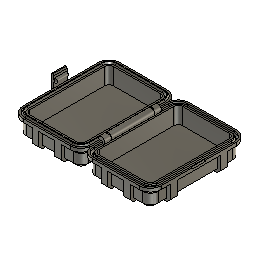
Parametric_Rugged_Box (Autodesk Fusion 360 design; units mm, degrees)
Autodesk Fusion 360 part; units mm, degrees
note: some values were not read from the file. Chosen so that the rebuilt part matches the saved one: where a step starts; which pieces of a blend or face edit are solid. Set by a fixed rule: which sketch regions a step uses.
sketch "Base Sketch" plane through (0, 0, 0) normal (0, 0, 1) x (1, 0, 0)
  line L0 (4, 0) -> (46, 0)
  line L1 (50, 4) -> (50, 71)
  line L2 (46, 75) -> (4, 75)
  line L3 (0, 71) -> (0, 4)
  arc A0 (46, 0) -> (50, 4) centre (46, 4) ccw
  arc A1 (50, 71) -> (46, 75) centre (46, 71) ccw
  arc A2 (4, 75) -> (0, 71) centre (4, 71) ccw
  arc A3 (0, 4) -> (4, 0) centre (4, 4) ccw
  point P0 (50, 0)
  point P1 (0, 75)
  dimension "d6" = 50
  dimension "d7" = 75
  dimension "d8" = 4
  constraint horizontal L0
  constraint vertical L1
  constraint horizontal L2
  constraint vertical L3
  constraint coincident P0 L0
  constraint coincident P0 L1
  constraint tangent L0 A0
  constraint tangent L1 A0
  constraint tangent L1 A1
  constraint tangent L2 A1
  constraint equal A0 A1
  constraint coincident P1 L2
  constraint coincident P1 L3
  constraint tangent L2 A2
  constraint tangent L3 A2
  constraint equal A0 A2
  constraint coincident origin L0
  constraint coincident origin L3
  constraint tangent L0 A3
  constraint tangent L3 A3
  constraint equal A0 A3
  measures "d6" distance of origin P0
  measures "d7" distance of origin P1
  measures "d8" radius of A0
ref_plane "WorkPlane1" through (0, 37.5, 0) normal (0, 1, 0) x (0, 0, 1)
sketch "Top Sketch" plane through (0, 37.5, 0) normal (0, 1, 0) x (1, 0, 0)
  line L0 (0, 0) -> (-3, 0)
  line L1 (-3, 0) -> (-3, -15)
  line L2 (-3, -15) -> (0, -15)
  line L3 (0, -15) -> (0, 0)
  line L4 (-3, -15) -> (-6, -15)
  line L5 (-6, -15) -> (-6, -12)
  line L6 (-6, -12) -> (-3, -12)
  line L7 (-3, -12) -> (-3, -15)
  line L8 (0, 0) -> (25, 0)
  line L9 (25, 0) -> (25, 3)
  line L10 (25, 3) -> (0, 3)
  line L11 (0, 3) -> (0, 0)
  line L12 (0, 3) -> (-3, 0)
  line L13 (-6, -12) -> (-3, -9)
  line L14 (-4.5, -15) -> (-3.3536, -16.1464)
  line L15 (-4.5, -15) -> (-2.3787, -15) construction
  line L16 (-2.6464, -16.1464) -> (-1.5, -15)
  arc A0 (-3.3536, -16.1464) -> (-2.6464, -16.1464) centre (-3, -15.7929) ccw
  dimension "d12" = 3
  dimension "d13" = 15
  dimension "d14" = 3
  dimension "d15" = 3
  dimension "d16" = 25
  dimension "d17" = 3
  dimension "d97" = 45
  dimension "d146" = 0.5
  dimension "d284" = 45
  constraint horizontal L0
  constraint vertical L1
  constraint horizontal L2
  constraint vertical L3
  constraint coincident L0.start L3.end
  constraint horizontal L4
  constraint vertical L5
  constraint horizontal L6
  constraint vertical L7
  constraint horizontal L8
  constraint vertical L9
  constraint horizontal L10
  constraint vertical L11
  constraint coincident L1 L13.end
  constraint parallel L12 L13
  constraint horizontal L15
  constraint midpoint L4 L14.start
  constraint midpoint L2 L16.end
  constraint tangent L14 A0
  constraint tangent L16 A0
  measures "d12" distance of L0.start L0.end
  measures "d13" distance of L0.start L2.end
  measures "d14" distance of L1.end L4.end
  measures "d15" distance of L1.end L6.end
  measures "d16" distance of L0.start L8.end
  measures "d17" distance of L0.start L10.end
  measures "d97" angle of L14 L15
  measures "d146" radius of A0
  measures "d284" angle of L2 L16
sweep "Sweep1" add profiles "Top Sketch" path "Base Sketch" along L0 A0 L1 A1 L2 A2 L3 A3 section 1 contours L0 L1 L2 L3 L7 | L8 L9 L10 L11 | L0 L11 L12 | L1 L6 L13 | L1 L4 L5 L6 L7 makes body 1
sketch "Bottom Sketch" plane through (0, 37.5, 0) normal (0, 1, 0) x (1, 0, 0)
  line L0 (0, 0) -> (-3, 0)
  line L1 (-3, 0) -> (-3, -15)
  line L2 (-3, -15) -> (0, -15)
  line L3 (0, -15) -> (0, 0)
  line L4 (0, 0) -> (25, 0)
  line L5 (25, 0) -> (25, 3)
  line L6 (25, 3) -> (0, 3)
  line L7 (0, 3) -> (0, 0)
  line L8 (-3, -15) -> (-6, -15)
  line L9 (-6, -15) -> (-6, -12)
  line L10 (-6, -12) -> (-3, -12)
  line L11 (-3, -12) -> (-3, -15)
  line L12 (0, 3) -> (-3, 0)
  line L13 (-6, -12) -> (-3, -9)
  line L14 (-4.5, -15) -> (-1.5, -15)
  line L15 (-1.5, -15) -> (-1.5, -12)
  line L16 (-1.5, -12) -> (-4.5, -12)
  line L17 (-4.5, -12) -> (-4.5, -15)
  line L18 (-3.3536, -12.3536) -> (-4.5, -13.5)
  line L19 (-2.6464, -12.3536) -> (-1.5, -13.5)
  arc A0 (-2.6464, -12.3536) -> (-3.3536, -12.3536) centre (-3, -12.7071) ccw
  dimension "d24" = 3
  dimension "d25" = 15
  dimension "d26" = 25
  dimension "d27" = 3
  dimension "d28" = 3
  dimension "d29" = 3
  dimension "d90" = 3
  dimension "d145" = 0.5
  constraint horizontal L0
  constraint vertical L1
  constraint horizontal L2
  constraint vertical L3
  constraint coincident L0.start L3.end
  constraint horizontal L4
  constraint vertical L5
  constraint horizontal L6
  constraint vertical L7
  constraint horizontal L8
  constraint vertical L9
  constraint horizontal L10
  constraint vertical L11
  constraint coincident L1 L13.end
  constraint parallel L12 L13
  constraint horizontal L14
  constraint vertical L15
  constraint horizontal L16
  constraint vertical L17
  constraint midpoint L8 L14.start
  constraint midpoint L17 L18.end
  constraint midpoint L15 L19.end
  constraint perpendicular L18 L19
  constraint coincident L10.end L18
  constraint coincident L10.end L19
  constraint tangent L18 A0
  constraint tangent L19 A0
  measures "d24" distance of L0.start L0.end
  measures "d25" distance of L0.start L2.end
  measures "d26" distance of L0.start L4.end
  measures "d27" distance of L0.start L6.end
  measures "d28" distance of L1.end L8.end
  measures "d29" distance of L1.end L10.end
  measures "d90" distance of L14.start L16.end
  measures "d145" radius of A0
sweep "Sweep2" add profiles "Bottom Sketch" path "Base Sketch" along L0 A0 L1 A1 L2 A2 L3 A3 section 1 separate body makes body 2
ref_plane "WorkPlane2" through (0, 18, 0) normal (0, 1, 0) x (0, 0, 1)
sketch "Rib Bottom" plane through (0, 18, 0) normal (0, 1, 0) x (1, 0, 0)
  line L0 (0, 0) -> (-6, 0)
  line L1 (-6, 0) -> (-6, -15)
  line L2 (-6, -15) -> (0, -15)
  line L3 (0, -15) -> (0, 0)
  line L4 (0, 0) -> (25, 0)
  line L5 (25, 0) -> (25, 3)
  line L6 (25, 3) -> (0, 3)
  line L7 (0, 3) -> (0, 0)
  line L8 (0, 0) -> (-3, 0)
  line L9 (-3, 0) -> (-3, 3)
  line L10 (-3, 3) -> (0, 3)
  line L11 (0, 3) -> (0, 0)
  line L12 (-3, 3) -> (-6, 0)
  dimension "d37" = 6
  dimension "d38" = 15
  dimension "d39" = 25
  dimension "d40" = 3
  dimension "d41" = 3
  dimension "d42" = 3
  constraint horizontal L0
  constraint vertical L1
  constraint horizontal L2
  constraint vertical L3
  constraint coincident L0.start L3.end
  constraint horizontal L4
  constraint vertical L5
  constraint horizontal L6
  constraint vertical L7
  constraint horizontal L8
  constraint vertical L9
  constraint horizontal L10
  constraint vertical L11
  measures "d37" distance of L0.start L0.end
  measures "d38" distance of L0.start L2.end
  measures "d39" distance of L0.start L4.end
  measures "d40" distance of L0.start L6.end
  measures "d41" distance of L0.start L8.end
  measures "d42" distance of L0.start L6.end
extrude "Extrude1" add sketch "Rib Bottom" against normal blind 6 bodies 2
ref_plane "WorkPlane3" through (0, 57, 0) normal (0, 1, 0) x (0, 0, 1)
extrude "Extrude2" add sketch "Rib Bottom" along normal blind 6 from surface at 39 bodies 2
ref_plane "WorkPlane4" through (25, 0, 0) normal (1, 0, 0) x (0, 1, 0)
mirror "Mirror1" about plane through (25, 0, 0) normal (1, 0, 0) of "Extrude1", "Extrude2"
sketch "Rib Top" plane through (0, 37.5, 0) normal (0, 1, 0) x (1, 0, 0)
  line L0 (0, 0) -> (-6, 0)
  line L1 (-6, 0) -> (-6, -15)
  line L2 (-6, -15) -> (0, -15)
  line L3 (0, -15) -> (0, 0)
  line L4 (0, 0) -> (25, 0)
  line L5 (25, 0) -> (25, 3)
  line L6 (25, 3) -> (0, 3)
  line L7 (0, 3) -> (0, 0)
  line L8 (0, 0) -> (-3, 0)
  line L9 (-3, 0) -> (-3, 3)
  line L10 (-3, 3) -> (0, 3)
  line L11 (0, 3) -> (0, 0)
  line L12 (-3, 3) -> (-6, 0)
  dimension "d52" = 6
  dimension "d53" = 15
  dimension "d54" = 25
  dimension "d55" = 3
  dimension "d56" = 3
  dimension "d57" = 3
  constraint horizontal L0
  constraint vertical L1
  constraint horizontal L2
  constraint vertical L3
  constraint coincident L0.start L3.end
  constraint horizontal L4
  constraint vertical L5
  constraint horizontal L6
  constraint vertical L7
  constraint horizontal L8
  constraint vertical L9
  constraint horizontal L10
  constraint vertical L11
  measures "d52" distance of L0.start L0.end
  measures "d53" distance of L0.start L2.end
  measures "d54" distance of L0.start L4.end
  measures "d55" distance of L0.start L6.end
  measures "d56" distance of L0.start L8.end
  measures "d57" distance of L0.start L6.end
extrude "Extrude3" add sketch "Rib Top" against normal blind 6 from surface at -19.5 bodies 1
extrude "Extrude4" add sketch "Rib Top" along normal blind 6 from surface at 19.5 bodies 1
mirror "Mirror2" about plane through (25, 0, 0) normal (1, 0, 0) of "Extrude3", "Extrude4"
ref_plane "WorkPlane5" through (18, 0, 0) normal (1, 0, 0) x (0, 1, 0)
ref_plane "WorkPlane6" through (32, 0, 0) normal (1, 0, 0) x (0, 1, 0)
sketch "Rib Wid" plane through (18, 0, 0) normal (1, 0, 0) x (0, 1, 0)
  line L0 (0, 0) -> (-6, 0)
  line L1 (-6, 0) -> (-6, 15)
  line L2 (-6, 15) -> (0, 15)
  line L3 (0, 15) -> (0, 0)
  line L4 (0, 0) -> (37.5, 0)
  line L5 (37.5, 0) -> (37.5, -3)
  line L6 (37.5, -3) -> (0, -3)
  line L7 (0, -3) -> (0, 0)
  line L8 (0, 0) -> (-3, 0)
  line L9 (-3, 0) -> (-3, -3)
  line L10 (-3, -3) -> (0, -3)
  line L11 (0, -3) -> (0, 0)
  line L12 (-3, -3) -> (-6, 0)
  line L13 (0, -3) -> (-6, -3)
  line L14 (-6, -3) -> (-6, 12)
  line L15 (-6, 12) -> (0, 12)
  line L16 (0, 12) -> (0, -3)
  dimension "d68" = 6
  dimension "d69" = 15
  dimension "d70" = 37.5
  dimension "d71" = 3
  dimension "d72" = 3
  dimension "d73" = 3
  dimension "d74" = 6
  dimension "d75" = 15
  constraint horizontal L0
  constraint vertical L1
  constraint horizontal L2
  constraint vertical L3
  constraint coincident L0.start L3.end
  constraint horizontal L4
  constraint vertical L5
  constraint horizontal L6
  constraint vertical L7
  constraint horizontal L8
  constraint vertical L9
  constraint horizontal L10
  constraint vertical L11
  constraint horizontal L13
  constraint vertical L14
  constraint horizontal L15
  constraint vertical L16
  measures "d68" distance of L0.start L0.end
  measures "d69" distance of L0.start L2.end
  measures "d70" distance of L0.start L4.end
  measures "d71" distance of L0.start L6.end
  measures "d72" distance of L0.start L8.end
  measures "d73" distance of L0.start L6.end
  measures "d74" distance of L6.end L13.end
  measures "d75" distance of L6.end L15.end
extrude "Extrude5" add sketch "Rib Wid" against normal blind 6 contours L0 L7 L8 L9 L10 L11 L13 L16 | L0 L1 L3 L8 L14 L15 L16 | L4 L5 L6 L7 L11 L16 | L0 L9 L12 | L1 L2 L3 L15 bodies 2
extrude "Extrude6" add sketch "Rib Wid" along normal blind 6 from surface at 14 contours L0 L7 L8 L9 L10 L11 L13 L16 | L0 L1 L3 L8 L14 L15 L16 | L4 L5 L6 L7 L11 L16 | L0 L9 L12 | L1 L2 L3 L15 bodies 2
ref_plane "WorkPlane7" through (25, 37.5, 4.5) normal (0, -1, 0) x (0, 0, -1)
mirror "Mirror3" about plane through (25, 37.5, 4.5) normal (0, -1, 0) of "Extrude5", "Extrude6"
extrude "Extrude7" add sketch "Rib Wid" against normal blind 6 contours L0 L7 L8 L9 L10 L11 L13 L16 | L0 L1 L3 L8 L14 L15 L16 | L4 L5 L6 L7 L11 L16 | L0 L9 L12 bodies 1
extrude "Extrude8" add sketch "Rib Wid" along normal blind 6 from surface at 14 contours L0 L7 L8 L9 L10 L11 L13 L16 | L0 L1 L3 L8 L14 L15 L16 | L4 L5 L6 L7 L11 L16 | L0 L9 L12 bodies 1
mirror "Mirror4" about plane through (25, 37.5, 4.5) normal (0, -1, 0) of "Extrude7", "Extrude8"
sweep "Sweep3" cut profiles "Bottom Sketch" path "Base Sketch" along L0 A0 L1 A1 L2 A2 L3 A3 section 1 contours L1 L2 L11 L14 L15 L19 A0 | L1 L8 L11 L14 L17 L18 A0 bodies 2
sweep "Sweep4" add profiles "Top Sketch" path "Base Sketch" along L0 A0 L1 A1 L2 A2 L3 A3 section 1 contours L2 L4 L14 L16 A0 bodies 1
sketch "Hinge" plane through (0, 0, 0) normal (0, 1, 0) x (1, 0, 0)
  line L0 (0, 0) -> (-6, 0) construction
  line L1 (-6, 0) -> (-6, -15) construction
  line L2 (-6, -15) -> (0, -15) construction
  line L3 (0, -15) -> (0, 0) construction
  circle A0 centre (-6, -15) radius 3
  circle A1 centre (-6, -15) radius 1.5
  circle A2 centre (-6, -15) radius 3.1
  line L4 (-6, -15) -> (-4.5, -15)
  line L5 (-4.5, -15) -> (-4.5, -18)
  line L6 (-4.5, -18) -> (-6, -18)
  line L7 (-6, -18) -> (-6, -15)
  line L8 (-6, -15) -> (-7.5, -15)
  line L9 (-7.5, -15) -> (-7.5, -18)
  line L10 (-7.5, -18) -> (-6, -18)
  line L11 (-6, -18) -> (-6, -15)
  line L12 (0, 0) -> (-6, 0) construction
  line L13 (-6, 0) -> (-6, -15) construction
  line L14 (-6, -15) -> (0, -15) construction
  line L15 (0, -15) -> (0, 0) construction
  circle A3 centre (-6, -15) radius 3
  circle A4 centre (-6, -15) radius 3.2
  dimension "d329" = 6
  dimension "d330" = 15
  dimension "d331" = 6
  dimension "d332" = 3
  dimension "d339" = 6.2
  dimension "d345" = 1.5
  dimension "d346" = 3
  dimension "d347" = 1.5
  dimension "d348" = 3
  dimension "d355" = 6
  dimension "d356" = 15
  dimension "d357" = 6
  dimension "d358" = 0.2
  constraint horizontal L0
  constraint vertical L1
  constraint horizontal L2
  constraint vertical L3
  constraint coincident L0.start L3.end
  constraint coincident L1.end L2.start
  constraint concentric A0 A1
  constraint concentric A0 A2
  constraint horizontal L4
  constraint vertical L5
  constraint horizontal L6
  constraint vertical L7
  constraint horizontal L8
  constraint vertical L9
  constraint horizontal L10
  constraint vertical L11
  constraint horizontal L12
  constraint vertical L13
  constraint horizontal L14
  constraint vertical L15
  measures "d329" distance of L0.start L0.end
  measures "d330" distance of L0.start L2.end
  measures "d331" diameter of A0
  measures "d332" diameter of A1
  measures "d339" diameter of A2
  measures "d345" distance of L1.end L4.end
  measures "d346" distance of L1.end L6.end
  measures "d347" distance of L1.end L8.end
  measures "d348" distance of L1.end L6.end
  measures "d355" distance of L0.start L0.end
  measures "d356" distance of L0.start L2.end
  measures "d357" diameter of A3
extrude "Extrude58" add sketch "Hinge" along normal up to surface (6 mm away) from surface at 12 contours A0 A1 L5 L9 A3 | A0 A1 L7 L9 L11 A3 | A0 A1 L5 L7 L11 A3 | A1 L7 L8 L11 | A1 L4 L8 | A1 L4 L7 L11 bodies 1
extrude "Extrude59" add sketch "Hinge" along normal up to surface (6 mm away) from surface at 57 contours A0 A1 L5 L9 A3 | A0 A1 L7 L9 L11 A3 | A0 A1 L5 L7 L11 A3 | A1 L7 L8 L11 | A1 L4 L8 | A1 L4 L7 L11 bodies 1
extrude "Extrude60" cut sketch "Hinge" along normal up to surface (39 mm away) from surface at 18 contours A0 A1 L5 L9 A3 | A0 A2 L5 L9 A3 | A0 A1 L7 L9 L11 A3 | A0 A2 L9 L10 A3 | A0 A2 L5 L6 A3 | A0 A1 L5 L7 L11 A3 | A2 L6 L10 | A1 L7 L8 L11 | A1 L4 L8 | A1 L4 L7 L11 bodies 1
extrude "Extrude61" cut sketch "Hinge" against normal blind 0.8 from surface at 18 contours A0 A1 L7 L9 L11 A3 | A0 A1 L5 L7 L11 A3 | A1 L7 L8 L11 | A1 L4 L7 L11 bodies 1
extrude "Extrude62" cut sketch "Hinge" along normal blind 0.8 from surface at 57 contours A0 A1 L7 L9 L11 A3 | A0 A1 L5 L7 L11 A3 | A1 L7 L8 L11 | A1 L4 L7 L11 bodies 1
extrude "Extrude63" cut sketch "Hinge" along normal up to surface (6.4 mm away) from surface at 11.8 contours A0 A1 L5 L9 A3 | A0 A2 L5 L9 A3 | A0 A1 L7 L9 L11 A3 | A0 A2 L9 L10 A3 | A0 A2 L5 L6 A3 | A0 A1 L5 L7 L11 A3 | A2 L6 L10 | A1 L7 L8 L11 | A1 L4 L8 | A2 L5 L9 A4 | A2 L9 L10 A4 | A1 L4 L7 L11 | A2 L5 L6 A4 | A2 L6 L10 A4 bodies 2
extrude "Extrude64" cut sketch "Hinge" along normal up to surface (6.4 mm away) from surface at 56.8 contours A0 A1 L5 L9 A3 | A0 A2 L5 L9 A3 | A0 A1 L7 L9 L11 A3 | A0 A2 L9 L10 A3 | A0 A2 L5 L6 A3 | A0 A1 L5 L7 L11 A3 | A2 L6 L10 | A1 L7 L8 L11 | A1 L4 L8 | A2 L5 L9 A4 | A2 L9 L10 A4 | A1 L4 L7 L11 | A2 L5 L6 A4 | A2 L6 L10 A4 bodies 2
extrude "Extrude65" add sketch "Hinge" along normal up to surface (38.6 mm away) from surface at 18.2 contours A0 A1 L5 L9 A3 | A0 A1 L7 L9 L11 A3 | A0 A1 L5 L7 L11 A3 | A1 L7 L8 L11 | A1 L4 L8 | A1 L4 L7 L11 bodies 2
sketch "Sketch16" plane through (0, 0, 0) normal (0, 1, 0) x (1, 0, 0)
  line L0 (0, 0) -> (50, 0) construction
  line L1 (50, 0) -> (50, -15) construction
  line L2 (50, -15) -> (0, -15) construction
  line L3 (0, -15) -> (0, 0) construction
  line L4 (50, 0) -> (51.5, 0) construction
  line L5 (51.5, 0) -> (51.5, -15) construction
  line L6 (51.5, -15) -> (50, -15) construction
  line L7 (50, -15) -> (50, 0) construction
  line L8 (51.5, -15) -> (54.5, -15)
  line L9 (54.5, -15) -> (54.5, -18)
  line L10 (54.5, -18) -> (51.5, -18)
  line L11 (51.5, -18) -> (51.5, -15)
  dimension "d370" = 50
  dimension "d371" = 15
  dimension "d372" = 1.5
  dimension "d373" = 15
  dimension "d374" = 3
  dimension "d375" = 3
  constraint horizontal L0
  constraint vertical L1
  constraint horizontal L2
  constraint vertical L3
  constraint coincident L0.start L3.end
  constraint horizontal L4
  constraint vertical L5
  constraint horizontal L6
  constraint vertical L7
  constraint horizontal L8
  constraint vertical L9
  constraint horizontal L10
  constraint vertical L11
  measures "d370" distance of L0.start L0.end
  measures "d371" distance of L0.start L2.end
  measures "d372" distance of L0.end L4.end
  measures "d373" distance of L0.end L1.end
  measures "d374" distance of L5.end L8.end
  measures "d375" distance of L5.end L10.end
sketch "Sketch17" plane through (0, 57, 0) normal (0, -1, 0) x (1, 0, 0)
  line L0 (-4.5, 17.5981) -> (-4.5, 15)
  line L1 (-4.5, 15) -> (-7.5, 15)
  line L2 (-7.5, 15) -> (-7.5, 17.5981)
  arc A0 (-7.5, 17.5981) -> (-6, 12) centre (-6, 15) ccw
  line L3 (-6, 12) -> (-6, 0)
  line L4 (-6, 0) -> (-3, -3)
  line L5 (-3, -3) -> (0, -3)
  line L6 (0, -3) -> (-3, 0)
  line L7 (-3, 0) -> (-3, 9)
  line L8 (-3, 9) -> (-5.9016, 11.9016)
  arc A1 (-5.9016, 11.9016) -> (-3.1691, 16.2634) centre (-6, 15) ccw
  arc A2 (-3.1691, 16.2634) -> (-3.2594, 16.2203) centre (-3, 15.7929) ccw
  arc A3 (-3.2594, 16.2203) -> (-4.5, 17.5981) centre (-6, 15) ccw
  circle A4 centre (-6, 15) radius 1.5
  dimension "d376" = 3
  constraint concentric A0 A4
  measures "d376" diameter of A4
revolve "Revolve1" cut sketch "Sketch17" angle 360 about axis through (-4.5, 57, 15) along (-1, 0, 0) contours L1 A4 picked at (-5.5166, 14.7781) bodies 1
sketch "Sketch18" plane through (0, 56.8, 0) normal (0, 1, 0) x (-1, 0, 0)
  line L0 (3.8787, 12.8787) -> (3.7373, 12.7373)
  arc A0 (3.7373, 12.7373) -> (5.8059, 11.8059) centre (6, 15) ccw
  line L1 (5.8059, 11.8059) -> (6, 12)
  arc A1 (6, 12) -> (3.8787, 12.8787) centre (6, 15) ccw
  circle A2 centre (6, 15) radius 1.5
  line L2 (6, 15) -> (4.5, 15)
  line L3 (6, 15) -> (6.2, 15)
  line L4 (6.2, 15) -> (7.5, 15)
  dimension "d378" = 3
  constraint concentric A0 A2
  constraint coincident A0.centre A1.centre
  constraint coincident A2 L2.end
  constraint horizontal L2
  constraint parallel L2 L3
  constraint coincident A2 L4.end
  constraint parallel L2 L4
  measures "d378" diameter of A2
revolve "Revolve2" add sketch "Sketch18" angle 360 about axis through (-6.2, 56.8, 15) along (-1, 0, 0) contours A2 L2 L3 L4 picked at (5.1364, 14.5014) bodies 2
sketch "Sketch19" plane through (0, 18.2, 0) normal (0, -1, 0) x (1, 0, 0)
  arc A0 (-3.8787, 12.8787) -> (-6, 12) centre (-6, 15) ccw
  line L0 (-6, 12) -> (-5.8059, 11.8059)
  arc A1 (-5.8059, 11.8059) -> (-3.7373, 12.7373) centre (-6, 15) ccw
  line L1 (-3.7373, 12.7373) -> (-3.8787, 12.8787)
  circle A2 centre (-6, 15) radius 1.5
  line L2 (-6, 15) -> (-4.5, 15)
  line L3 (-6, 15) -> (-7.5, 15)
  dimension "d380" = 3
  constraint concentric A0 A2
  constraint coincident A0.centre A1.centre
  constraint coincident A2 L2.end
  constraint horizontal L2
  constraint coincident A2 L3.end
  constraint parallel L2 L3
  measures "d380" diameter of A2
revolve "Revolve3" add sketch "Sketch19" angle 360 about axis through (-6, 18.2, 15) along (1, 0, 0) contours A2 L2 L3 picked at (-5.0056, 14.9255) bodies 2
sketch "Sketch20" plane through (0, 18, 0) normal (0, 1, 0) x (-1, 0, 0)
  line L0 (4.5, 15) -> (4.5, 17.5981)
  arc A0 (4.5, 17.5981) -> (3.2594, 16.2203) centre (6, 15) ccw
  arc A1 (3.2594, 16.2203) -> (3.1691, 16.2634) centre (3, 15.7929) ccw
  arc A2 (3.1691, 16.2634) -> (5.9016, 11.9016) centre (6, 15) ccw
  line L1 (5.9016, 11.9016) -> (3, 9)
  line L2 (3, 9) -> (3, 0)
  line L3 (3, 0) -> (0, -3)
  line L4 (0, -3) -> (3, -3)
  line L5 (3, -3) -> (6, 0)
  line L6 (6, 0) -> (6, 12)
  arc A3 (6, 12) -> (7.5, 17.5981) centre (6, 15) ccw
  line L7 (7.5, 17.5981) -> (7.5, 15)
  line L8 (7.5, 15) -> (4.5, 15)
  circle A4 centre (6, 15) radius 1.5
  dimension "d382" = 3
  constraint concentric A0 A4
  measures "d382" diameter of A4
revolve "Revolve4" cut sketch "Sketch20" angle 360 about axis through (-7.5, 18, 15) along (1, 0, 0) contours L8 A4 picked at (6.5647, 14.571) bodies 1
chamfer "Chamfer10" distance 0.79 angle 45 4 edges at (-4.5, 57.8, 16.299) (-7.5, 57.8, 16.299) (-4.5, 17.2, 16.299) (-7.5, 17.2, 16.299) on bodies 1
sketch "Latch" plane through (0, 0, 0) normal (0, 1, 0) x (1, 0, 0)
  line L0 (0, 0) -> (53, 0) construction
  line L1 (53, 0) -> (53, -15) construction
  line L2 (53, -15) -> (0, -15) construction
  line L3 (0, -15) -> (0, 0) construction
  line L4 (0, 0) -> (53, 0) construction
  line L5 (53, 0) -> (53, -15)
  line L6 (53, -15) -> (0, -15) construction
  line L7 (0, -15) -> (0, 0) construction
  line L8 (53, -15) -> (56, -15) construction
  line L9 (56, -15) -> (56, -12) construction
  line L10 (56, -12) -> (53, -12) construction
  line L11 (53, -12) -> (53, -15) construction
  line L12 (53, -15) -> (56, -15) construction
  line L13 (56, -15) -> (56, -12) construction
  line L14 (56, -12) -> (53, -12) construction
  line L15 (53, -12) -> (53, -15) construction
  line L16 (53, -12) -> (56, -12)
  line L17 (56, -12) -> (56, -9)
  line L18 (56, -9) -> (53, -9)
  line L19 (53, -9) -> (53, -12)
  line L20 (53, -12) -> (56, -12)
  line L21 (56, -12) -> (56, -9)
  line L22 (56, -9) -> (53, -9)
  line L23 (53, -9) -> (53, -12)
  line L24 (56, -12) -> (59, -12)
  line L25 (59, -12) -> (59, -20.5)
  line L26 (59, -20.5) -> (56, -20.5)
  line L27 (56, -20.5) -> (56, -12)
  line L28 (53, -15) -> (56, -15)
  line L29 (56, -15) -> (56, -18)
  line L30 (56, -18) -> (53, -18)
  line L31 (53, -18) -> (53, -15)
  line L32 (59, -12) -> (56, -9)
  circle A0 centre (56, -20.5) radius 2
  line L33 (56, -9) -> (53, -6)
  line L34 (56, -9) -> (80.2426, -9) construction
  dimension "d385" = 53
  dimension "d386" = 15
  dimension "d387" = 53
  dimension "d388" = 15
  dimension "d389" = 3
  dimension "d390" = 3
  dimension "d391" = 3
  dimension "d392" = 3
  dimension "d393" = 3
  dimension "d394" = 3
  dimension "d395" = 3
  dimension "d396" = 3
  dimension "d397" = 3
  dimension "d398" = 8.5
  dimension "d399" = 3
  dimension "d400" = 3
  dimension "d401" = 4
  dimension "d402" = 135
  constraint horizontal L0
  constraint vertical L1
  constraint horizontal L2
  constraint vertical L3
  constraint coincident L0.start L3.end
  constraint horizontal L4
  constraint vertical L5
  constraint horizontal L6
  constraint vertical L7
  constraint horizontal L8
  constraint vertical L9
  constraint horizontal L10
  constraint vertical L11
  constraint horizontal L12
  constraint vertical L13
  constraint horizontal L14
  constraint vertical L15
  constraint horizontal L16
  constraint vertical L17
  constraint horizontal L18
  constraint vertical L19
  constraint horizontal L20
  constraint vertical L21
  constraint horizontal L22
  constraint vertical L23
  constraint horizontal L24
  constraint vertical L25
  constraint horizontal L26
  constraint vertical L27
  constraint horizontal L28
  constraint vertical L29
  constraint horizontal L30
  constraint vertical L31
  constraint horizontal L34
  constraint coincident L1 L33.end
  constraint coincident L26.end L27.start
  measures "d385" distance of L0.start L0.end
  measures "d386" distance of L0.start L2.end
  measures "d387" distance of L0.start L0.end
  measures "d388" distance of L0.start L2.end
  measures "d389" distance of L1.end L8.end
  measures "d390" distance of L1.end L10.end
  measures "d391" distance of L1.end L8.end
  measures "d392" distance of L1.end L10.end
  measures "d393" distance of L10.end L9.end
  measures "d394" distance of L10.end L18.end
  measures "d395" distance of L10.end L9.end
  measures "d396" distance of L10.end L18.end
  measures "d397" distance of L9.end L24.end
  measures "d398" distance of L9.end L26.end
  measures "d399" distance of L1.end L8.end
  measures "d400" distance of L1.end L30.end
  measures "d401" diameter of A0
  measures "d402" angle of L33 L34
extrude "Extrude66" add sketch "Latch" along normal mid plane 12 from surface at 37.5 contours L5 L18 L22 L33 | L5 L16 L17 L18 L19 L20 L21 L22 L23 | L17 L21 L24 L32 | L24 L25 L26 L27 L29 A0 | L26 L27 A0 | L26 L27 A0 bodies 1
extrude "Extrude67" cut sketch "Latch" along normal mid plane 12.8 from surface at 37.5 contours L5 L16 L17 L18 L19 L20 L21 L22 L23 bodies 2
chamfer "Chamfer11" distance 2 angle 45 2 edges at (54.5, 43.9, 10.5) (54.5, 31.1, 10.5) on bodies 2
chamfer "Chamfer12" distance 1 angle 45 4 edges at (54.5858, 31.5, 21.9142) (59, 31.5, 16.25) (54.5858, 43.5, 21.9142) (59, 43.5, 16.25) on bodies 1
sketch "Sketch22" plane through (0, 31.5, 0) normal (0, -1, 0) x (1, 0, 0)
  line L0 (58, 11) -> (58, 20.5)
  arc A0 (57, 20.5) -> (56, 19.5) centre (56, 20.5) ccw
  line L1 (56, 19.5) -> (56, 15)
  line L2 (56, 15) -> (56, 12)
  line L3 (56, 12) -> (53, 9)
  line L4 (56, 19.5) -> (59, 19.5)
  line L5 (59, 19.5) -> (59, 25.5)
  line L6 (59, 25.5) -> (56, 25.5)
  line L7 (56, 25.5) -> (56, 19.5)
  line L8 (58, 20.5) -> (57, 20.5)
  line L9 (53, 9) -> (53, 6)
  line L10 (53, 6) -> (58, 11)
  dimension "d412" = 3
  dimension "d413" = 6
  constraint horizontal L4
  constraint vertical L5
  constraint horizontal L6
  constraint vertical L7
  constraint coincident A0.end L1.start
  measures "d412" distance of A0.end L4.end
  measures "d413" distance of A0.end L6.end
extrude "Extrude68" add sketch "Sketch22" against normal blind 12 contours L0 A0 L4 L7 L8 | L0 A0 L4 L5 L6 L7 L8 bodies 1
chamfer "Chamfer14" distance 1 angle 45 2 edges at (59, 31.5, 22.5) (59, 43.5, 22.5) on bodies 1
chamfer "Chamfer15" distance 1 angle 45 2 edges at (59, 37.5, 25.5) (56, 37.5, 25.5) on bodies 1
copy_body "Body->Comp1" bodies 1 removing the originals makes body 3 in component "Top"
copy_body "Body->Comp2" bodies 2 removing the originals makes body 4 in component "Bottom"
sketch "Sketch23" plane through (56, 0, 0) normal (1, 0, 0) x (0, 1, 0)
  line L0 (63, 37) -> (71, 37)
  line L1 (71, 37) -> (71, 40)
  line L2 (71, 40) -> (4, 40)
  line L3 (4, 40) -> (4, 37)
  line L4 (4, 37) -> (12, 37)
  line L5 (12, 37) -> (12, 25)
  line L6 (12, 25) -> (18, 25)
  line L7 (18, 25) -> (18, 37)
  line L8 (18, 37) -> (29.1, 37)
  line L9 (29.1, 37) -> (45.9, 37)
  line L10 (45.9, 37) -> (57, 37)
  line L11 (57, 37) -> (57, 25)
  line L12 (57, 25) -> (63, 25)
  line L13 (63, 25) -> (63, 37)
  line L14 (37.5, 40) -> (43.7, 40)
  line L15 (37.5, 40) -> (31.3, 40)
  line L16 (31.3, 40) -> (43.7, 40)
  line L17 (43.7, 40) -> (43.7, 39.5)
  line L18 (43.7, 39.5) -> (31.3, 39.5)
  line L19 (31.3, 39.5) -> (31.3, 40)
  dimension "d423" = 6.2
  dimension "d424" = 6.2
  dimension "d425" = 0.5
  constraint midpoint L2 L14.start
  constraint parallel L2 L14
  constraint parallel L2 L15
  constraint horizontal L16
  constraint vertical L17
  constraint horizontal L18
  constraint vertical L19
  measures "d423" distance of L14.start L14.end
  measures "d424" distance of L14.start L15.end
  measures "d425" distance of L15.end L18.end
extrude "Extrude1'" cut sketch "Sketch23" against normal blind 1 contours L2 L14 L15 L16 L17 L18 L19 sketch seen with x (1, 0, 0) y (0, 1, 0) z (0, 0, 1) at (0, 0, -25) bodies 4 in component "Bottom"
extrude "Extrude2'" cut 1 faces at (55.3333, 39.5667, 14.5) along direction (0, 0, -1) blind 0.5 on bodies 4 bodies 4 in component "Bottom"
chamfer "Chamfer1" distance 1 angle 45 1 edges at (55, 37.5, 14) on bodies 4 in component "Bottom"
chamfer "Chamfer2" distance 0.7 angle 45 2 edges at (55.5, 31.3, 14.5) (55.5, 43.7, 14.5) on bodies 4 in component "Bottom"
chamfer "Chamfer1'" distance 1 angle 45 2 edges at (55.5, 31.5, 8.5) (55.5, 43.5, 8.5) on bodies 3 in component "Top"
component "Top" placed x (-1, 0, 0) y (0, -1, 0) z (0, 0, 1) at (-12, 75, 25)
component "Bottom" placed x (1, 0, 0) y (0, 1, 0) z (0, 0, 1) at (0, 0, 25)
equation "len = 75 mm" comment "Min 50mm"
equation "wid = 50 mm" comment "Min 30mm"
equation "hei = 30 mm" comment "Min 15mm if split .5; Min 30 if split .25"
equation "shell = 3 mm" comment "Don't change. This is used in a lot of calculations"
equation "fillet = 4 mm" comment "Controls curvature of corners"
equation "d6 = wid"
equation "d7 = len"
equation "d8 = fillet"
equation "d9 = len / 2"
equation "splitTop = hei * 0.5" comment "Determines % of internal dimensions is within the lid"
equation "splitBottom = hei - splitTop" comment "Don't change"
equation "d12 = shell"
equation "d13 = splitTop"
equation "d14 = shell"
equation "d15 = shell"
equation "d16 = wid / 2"
equation "d17 = shell"
equation "d24 = shell"
equation "d25 = splitBottom"
equation "d26 = wid / 2"
equation "d27 = shell"
equation "d28 = shell"
equation "d29 = shell"
equation "d36 = shell * 6"
equation "d37 = shell * 2"
equation "d38 = splitBottom"
equation "d39 = wid / 2"
equation "d40 = shell"
equation "d41 = shell"
equation "d42 = shell"
equation "d43 = -shell * 2"
equation "d45 = len - ( shell * 6 )"
equation "d47 = shell * 2"
equation "d49 = wid / 2"
equation "d52 = shell * 2"
equation "d53 = splitTop"
equation "d54 = wid / 2"
equation "d55 = shell"
equation "d56 = shell"
equation "d57 = shell"
equation "d59 = -shell * 2"
equation "d62 = shell * 2"
equation "d66 = shell * 6"
equation "d67 = wid - ( shell * 6 )"
equation "d68 = shell * 2"
equation "d69 = splitBottom"
equation "d70 = len / 2"
equation "d71 = shell"
equation "d72 = shell"
equation "d73 = shell"
equation "d74 = shell * 2"
equation "d75 = splitTop"
equation "d76 = -shell * 2"
equation "d79 = shell * 2"
equation "d83 = -shell * 2"
equation "d86 = shell * 2"
equation "d90 = shell"
equation "clearance = 0.2 mm" comment "Don't change"
equation "d329 = shell * 2"
equation "d330 = splitTop"
equation "d331 = shell * 2"
equation "d332 = shell"
equation "d339 = shell * 2 + clearance"
equation "d345 = shell / 2"
equation "d346 = shell"
equation "d347 = shell / 2"
equation "d348 = shell"
equation "d350 = -clearance * 4"
equation "d353 = clearance * 4"
equation "d355 = shell * 2"
equation "d356 = splitBottom"
equation "d357 = shell * 2"
equation "d358 = clearance"
equation "d359 = clearance"
equation "d360 = clearance"
equation "d362 = clearance"
equation "d363 = clearance"
equation "d370 = wid"
equation "d371 = splitTop"
equation "d372 = shell / 2"
equation "d373 = splitTop"
equation "d374 = shell"
equation "d375 = shell"
equation "d376 = shell"
equation "d378 = shell"
equation "d380 = shell"
equation "d382 = shell"
equation "d385 = wid + shell"
equation "d386 = splitTop"
equation "d387 = wid + shell"
equation "d388 = splitBottom"
equation "d389 = shell"
equation "d390 = shell"
equation "d391 = shell"
equation "d392 = shell"
equation "d393 = shell"
equation "d394 = shell"
equation "d395 = shell"
equation "d396 = shell"
equation "d397 = shell"
equation "d398 = shell * 3 - 0.5 mm"
equation "d399 = shell"
equation "d400 = shell"
equation "d401 = shell * 2 - 2 mm"
equation "d404 = shell * 2"
equation "d407 = shell * 2 + ( clearance * 2 )"
equation "d412 = shell"
equation "d413 = shell * 2"
equation "d421 = -clearance"
equation "d423 = shell * 2 + clearance"
equation "d424 = shell * 2 + clearance"
named bodies: "Top", "Bottom"
